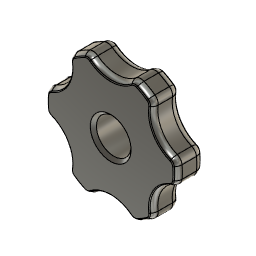
[a]_Thumb_Nut_x3 (Autodesk Fusion 360 design; units mm, degrees)
Autodesk Fusion 360 part; units mm, degrees
sketch "Sketch1" plane through (0, 0, 0) normal (0, 1, 0) x (1, 0, 0) in component "[a]_Thumb_Nut_x3"
  circle A0 centre (0, 0) radius 8.5
  arc A1 (-3.5191, -7.7373) -> (-2.484, -7.6109) centre (-3.1051, -6.8271) ccw
  arc A2 (0, -6.7461) -> (-2.484, -7.6109) centre (0, -10.7461) ccw
  line L0 (0, 0) -> (0, -11) construction
  arc A3 (2.484, -7.6109) -> (3.5191, -7.7373) centre (3.1051, -6.8271) ccw
  arc A4 (2.484, -7.6109) -> (0, -6.7461) centre (0, -10.7461) ccw
  arc A5 (4.9412, -6.9163) -> (5.3492, -5.9567) centre (4.3599, -6.1026) ccw
  arc A6 (5.8423, -3.373) -> (5.3492, -5.9567) centre (9.3064, -5.373) ccw
  arc A7 (7.8332, -1.6542) -> (5.8423, -3.373) centre (9.3064, -5.373) ccw
  arc A8 (7.8332, -1.6542) -> (8.4603, -0.8211) centre (7.4649, -0.7245) ccw
  arc A9 (8.4603, 0.8211) -> (7.8332, 1.6542) centre (7.4649, 0.7245) ccw
  arc A10 (5.8423, 3.373) -> (7.8332, 1.6542) centre (9.3064, 5.373) ccw
  arc A11 (5.3492, 5.9567) -> (5.8423, 3.373) centre (9.3064, 5.373) ccw
  arc A12 (5.3492, 5.9567) -> (4.9412, 6.9163) centre (4.3599, 6.1026) ccw
  arc A13 (3.5191, 7.7373) -> (2.484, 7.6109) centre (3.1051, 6.8271) ccw
  arc A14 (0, 6.7461) -> (2.484, 7.6109) centre (0, 10.7461) ccw
  arc A15 (-2.484, 7.6109) -> (0, 6.7461) centre (0, 10.7461) ccw
  arc A16 (-2.484, 7.6109) -> (-3.5191, 7.7373) centre (-3.1051, 6.8271) ccw
  arc A17 (-4.9412, 6.9163) -> (-5.3492, 5.9567) centre (-4.3599, 6.1026) ccw
  arc A18 (-5.8423, 3.373) -> (-5.3492, 5.9567) centre (-9.3064, 5.373) ccw
  arc A19 (-7.8332, 1.6542) -> (-5.8423, 3.373) centre (-9.3064, 5.373) ccw
  arc A20 (-7.8332, 1.6542) -> (-8.4603, 0.8211) centre (-7.4649, 0.7245) ccw
  arc A21 (-8.4603, -0.8211) -> (-7.8332, -1.6542) centre (-7.4649, -0.7245) ccw
  arc A22 (-5.8423, -3.373) -> (-7.8332, -1.6542) centre (-9.3064, -5.373) ccw
  arc A23 (-5.3492, -5.9567) -> (-5.8423, -3.373) centre (-9.3064, -5.373) ccw
  arc A24 (-5.3492, -5.9567) -> (-4.9412, -6.9163) centre (-4.3599, -6.1026) ccw
  dimension "d1" = 17
  dimension "d3" = 1
  dimension "d4" = 4
  dimension "d6" = 360
  constraint coincident A0.centre L0.start
  constraint coincident A0 A1.start
  constraint vertical L0
  constraint tangent A1 A2
  constraint coincident A2.start L0
  constraint coincident A2.centre L0
  constraint tangent A0 A1
  constraint symmetric A1.start L0 A3.end
  constraint symmetric A1.end L0 A3.start
  constraint symmetric A1 L0 A3
  constraint symmetric A2.start L0 A4.end
  constraint symmetric A2 L0 A4
  measures "d1" diameter of A0
  measures "d3" radius of A1
  measures "d4" radius of A2
extrude "Extrude1" add sketch "Sketch1" along normal blind 3.5 contours A0 A1 A2 A3 A4 A5 A6 A7 A8 A9 A10 A11 A12 A13 A14 A15 A16 A17 A18 A19 A20 A21 A22 A23 A24 in component "[a]_Thumb_Nut_x3"
sketch "Sketch2" plane through (0, 0, 0) normal (1, 0, 0) x (0, 1, 0) in component "[a]_Thumb_Nut_x3"
  arc A0 (3.5, 5.9921) -> (4, 5.126) centre (4.5, 5.9921) ccw
  arc A1 (4.5, 4.26) -> (4, 5.126) centre (3.5, 4.26) ccw
  line L0 (3.5, 4.26) -> (4.8882, 4.26) construction
  line L1 (4.5, 5.9921) -> (3.3446, 5.9921) construction
  line L2 (0, 7.6109) -> (0, 7.8271) construction
  line L3 (0, 7.7373) -> (3.5, 7.7373) construction
  line L4 (3.5, 7.6109) -> (3.5, 7.8271) construction
  line L5 (3.5, 7.6109) -> (0, 7.6109) construction
  line L6 (3.5, -0.8211) -> (3.5, 0.8211)
  line L7 (4.5, 4.26) -> (4.5, 0)
  line L8 (4.5, 0) -> (3.5, 0)
  line L9 (3.5, 5.9921) -> (3.5, 0)
  dimension "d9" = 1
  dimension "d10" = 1
  dimension "d12" = 1
  dimension "d13" = 4.26
  constraint tangent A0 A1
  constraint coincident A1.centre L0.start
  constraint horizontal L0
  constraint coincident A1.start L0
  constraint coincident A0.centre L1.start
  constraint horizontal L1
  constraint coincident A0.start L1
  constraint coincident A0.start L6
  constraint tangent A1 L7
  constraint midpoint L6 L8.end
  constraint perpendicular L6 L8
  measures "d9" radius of A0
  measures "d10" radius of A1
  measures "d12" horizontal distance of A0.start A1.start
  measures "d13" vertical distance of origin A1.centre
revolve "Revolve1" add sketch "Sketch2" angle 360 about axis through (0, 1.75, 0) along (0, 1, 0) in component "[a]_Thumb_Nut_x3"
hole "Hole1" at (0, 0, 0) direction (0, 1, 0) diameter 4.5 end through all in component "[a]_Thumb_Nut_x3"
chamfer "Chamfer1" distance 0.4 angle 45 1 faces at (0.1122, 1.5, -2.2472) in component "[a]_Thumb_Nut_x3"
chamfer "Chamfer2" distance 0.4 angle 45 48 edges at (0, 0, 6.7461) (-2.9838, 0, 7.8197) (-4.25, 0, 7.3612) (-5.2802, 0, 6.4938) (-5.8423, 0, 3.373) (-8.2639, 0, 1.3258) (-8.5, 0, 0) (-8.2639, 0, -1.3258) (-5.8423, 0, -3.373) (-5.2802, 0, -6.4938) (-4.25, 0, -7.3612) (-2.9838, 0, -7.8197) (0, 0, -6.7461) (2.9838, 0, -7.8197) (4.25, 0, -7.3612) (5.2802, 0, -6.4938) (5.8423, 0, -3.373) (8.2639, 0, -1.3258) (8.5, 0, 0) (8.2639, 0, 1.3258) (5.8423, 0, 3.373) (5.2802, 0, 6.4938) (4.25, 0, 7.3612) (2.9838, 0, 7.8197) (4.25, 3.5, 7.3612) (5.2802, 3.5, 6.4938) (5.8423, 3.5, 3.373) (8.2639, 3.5, 1.3258) (8.5, 3.5, 0) (8.2639, 3.5, -1.3258) (5.8423, 3.5, -3.373) (5.2802, 3.5, -6.4938) (4.25, 3.5, -7.3612) (2.9838, 3.5, -7.8197) (0, 3.5, -6.7461) (-2.9838, 3.5, -7.8197) (-4.25, 3.5, -7.3612) (-5.2802, 3.5, -6.4938) (-5.8423, 3.5, -3.373) (-8.2639, 3.5, -1.3258) (-8.5, 3.5, 0) (-8.2639, 3.5, 1.3258) (-5.8423, 3.5, 3.373) (-5.2802, 3.5, 6.4938) (-4.25, 3.5, 7.3612) (-2.9838, 3.5, 7.8197) (0, 3.5, 6.7461) (2.9838, 3.5, 7.8197) measured on face at (-2.6522, 0, 4.7258) measured on face at (-3.0292, 2.3333, 7.8242) measured on face at (-3.6846, 2.3333, 7.6599) measured on face at (-5.3359, 2.3333, 6.32) measured on face at (-2.6522, 0, 4.7258) measured on face at (-8.1069, 2.3333, 1.4912) measured on face at (-8.4877, 1.1667, 0.4566) measured on face at (-8.1413, 2.3333, -1.4611) measured on face at (-2.6522, 0, 4.7258) measured on face at (-5.312, 2.3333, -6.4082) measured on face at (-4.7914, 2.3333, -7.0209) measured on face at (-2.6777, 2.3333, -7.7312) measured on face at (-2.6522, 0, 4.7258) measured on face at (2.5582, 2.3333, -7.6643) measured on face at (4.7914, 1.1667, -7.0209) measured on face at (5.3359, 2.3333, -6.32) measured on face at (-2.6522, 0, 4.7258) measured on face at (8.1069, 2.3333, -1.4912) measured on face at (8.4995, 1.1667, 0.0914) measured on face at (8.0343, 2.3333, 1.5466) measured on face at (-2.6522, 0, 4.7258) measured on face at (5.3592, 2.3333, 6.139) measured on face at (4.3289, 2.3333, 7.3151) measured on face at (2.8053, 2.3333, 7.7811) measured on face at (-2.8677, 3.5, 6.9156) measured on face at (-2.8677, 3.5, 6.9156) measured on face at (-2.8677, 3.5, 6.9156) measured on face at (-2.8677, 3.5, 6.9156) measured on face at (-2.8677, 3.5, 6.9156) measured on face at (-2.8677, 3.5, 6.9156) measured on face at (-2.8677, 3.5, 6.9156) measured on face at (-2.8677, 3.5, 6.9156) measured on face at (-2.8677, 3.5, 6.9156) measured on face at (-2.8677, 3.5, 6.9156) measured on face at (-2.8677, 3.5, 6.9156) measured on face at (-2.8677, 3.5, 6.9156) measured on face at (-2.8677, 3.5, 6.9156) measured on face at (-2.8677, 3.5, 6.9156) measured on face at (-2.8677, 3.5, 6.9156) measured on face at (-2.8677, 3.5, 6.9156) measured on face at (-2.8677, 3.5, 6.9156) measured on face at (-2.8677, 3.5, 6.9156) measured on face at (-2.8677, 3.5, 6.9156) measured on face at (-2.8677, 3.5, 6.9156) measured on face at (-2.8677, 3.5, 6.9156) measured on face at (-2.8677, 3.5, 6.9156) measured on face at (-2.8677, 3.5, 6.9156) measured on face at (-2.8677, 3.5, 6.9156) in component "[a]_Thumb_Nut_x3"
fillet "Fillet1" radius 1 48 edges at (0, 0.4, 6.7461) (-2.9838, 0.4, 7.8197) (-4.25, 0.4, 7.3612) (-5.2802, 0.4, 6.4938) (-5.8423, 0.4, 3.373) (-8.2639, 0.4, 1.3258) (-8.5, 0.4, 0) (-8.2639, 0.4, -1.3258) (-5.8423, 0.4, -3.373) (-5.2802, 0.4, -6.4938) (-4.25, 0.4, -7.3612) (-2.9838, 0.4, -7.8197) (0, 0.4, -6.7461) (2.9838, 0.4, -7.8197) (4.25, 0.4, -7.3612) (5.2802, 0.4, -6.4938) (5.8423, 0.4, -3.373) (8.2639, 0.4, -1.3258) (8.5, 0.4, 0) (8.2639, 0.4, 1.3258) (5.8423, 0.4, 3.373) (5.2802, 0.4, 6.4938) (4.25, 0.4, 7.3612) (2.9838, 0.4, 7.8197) (5.8423, 3.1, 3.373) (8.2639, 3.1, 1.3258) (8.5, 3.1, 0) (8.2639, 3.1, -1.3258) (5.8423, 3.1, -3.373) (5.2802, 3.1, -6.4938) (4.25, 3.1, -7.3612) (2.9838, 3.1, -7.8197) (0, 3.1, -6.7461) (-2.9838, 3.1, -7.8197) (-4.25, 3.1, -7.3612) (-5.2802, 3.1, -6.4938) (-5.8423, 3.1, -3.373) (-8.2639, 3.1, -1.3258) (-8.5, 3.1, 0) (-8.2639, 3.1, 1.3258) (-5.8423, 3.1, 3.373) (-5.2802, 3.1, 6.4938) (-4.25, 3.1, 7.3612) (-2.9838, 3.1, 7.8197) (0, 3.1, 6.7461) (2.9838, 3.1, 7.8197) (4.25, 3.1, 7.3612) (5.2802, 3.1, 6.4938) in component "[a]_Thumb_Nut_x3"
component "[a]_Thumb_Nut_x3" placed x (1, 0, 0) y (0, 1, 0) z (0, 0, 1) at (0, -1.9785, 0)
